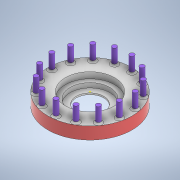
# Autodesk Inventor part: Część1
Saved by Autodesk Inventor 2021 (Build 250183000, 183)
## iProperties
Created: 2022-07-15
Part Number: Część1
Material: Ogólny
Document SubType Name: Modeling
Designer: MicnedSQ
Density: 1 g/cm^3
Appearance: Domyślna
Author: MicnedSQ
## iProperties of the stored document _Drukowanie 3D.ipt
Created: 2022-08-08
Part Number: _Drukowanie 3D
Material: Ogólny
Document SubType Name: Modeling
Designer: MicnedSQ
Density: 1 g/cm^3
Appearance: Domyślna
Author: MicnedSQ
Autodesk Inventor part; units mm, degrees
ref_plane "YZ Plane" through (0, 0, 0) normal (1, 0, 0) x (0, 1, 0)
ref_plane "XZ Plane" through (0, 0, 0) normal (0, 1, 0) x (-1, 0, 0)
ref_plane "XY Plane" through (0, 0, 0) normal (0, 0, 1) x (1, 0, 0)
sketch "Szkic1" plane through (0, 0, 0) normal (0, 1, 0) x (-1, 0, 0)
  circle A0 centre (0, 0) radius 27.5
  dimension "d0" = 55
  constraints: 1 centre point, 1 coincident
  measures "d0" diameter of A0
extrude "Wyciągnięcie proste1" add sketch "Szkic1" along normal blind 8
sketch "Szkic2" plane through (0, 8, 0) normal (0, 1, 0) x (1, 0, 0)
  circle A0 centre (0, 0) radius 25
  circle A1 centre (-25, 0) radius 1.5
  dimension "d3" = 50
  dimension "d4" = 3
  constraints: 1 centre point, 1 coincident, 1 horizontal alignment, 2 other
  measures "d4" diameter of A1
extrude "Wyciągnięcie proste2" add sketch "Szkic2" along normal blind 10 contours A1 A0 | A0 A1 picked at (-24.4967, 0) picked at (-25.4929, -0.0614)
pattern_circular "Szyk kołowy1" count 15 over 360 about axis through (0, 0, 0) along (0, 1, 0) of "Wyciągnięcie proste2"
sketch "Szkic4" plane through (0, 8, 0) normal (0, 1, 0) x (1, 0, 0)
  point P0 (0, 0)
sketch "Szkic5" plane through (0, 8, 0) normal (0, 1, 0) x (1, 0, 0)
  circle A0 centre (0, 0) radius 16.1
  dimension "d13" = 32.2
  constraints: 1 centre point, 1 coincident
  measures "d13" diameter of A0
extrude "Wyciągnięcie proste4" cut sketch "Szkic5" against normal blind 4
sketch "Szkic6" plane through (0, 4, 0) normal (0, 1, 0) x (1, 0, 0)
  circle A0 centre (0, 0) radius 13
  dimension "d16" = 26
  constraints: 1 centre point, 1 coincident
  measures "d16" diameter of A0
extrude "Wyciągnięcie proste5" cut sketch "Szkic6" against normal blind 3
sketch "Szkic9" plane through (0, 0, 0) normal (0, -1, 0) x (1, 0, 0)
  circle A0 centre (24, 0) radius 2.05
  circle A1 centre (0, 24) radius 2.05
  circle A2 centre (-24, 0) radius 2.05
  circle A3 centre (0, -24) radius 2.05
  point P0 (0, 0)
  dimension "d23" = 4.1
  dimension "d26" = 360
  dimension "d30" = 24
  constraints: 4 centre point, 9 other
  measures "d23" diameter of A0
  measures "d30" distance of point (0, 0) A0.centre
extrude "Wyciągnięcie proste7" cut sketch "Szkic9" against normal blind 7
sketch "Szkic10" plane through (0, 1, 0) normal (0, 1, 0) x (1, 0, 0)
  circle A0 centre (0, 0) radius 9
  dimension "d32" = 18
  constraints: 1 centre point, 1 coincident
  measures "d32" diameter of A0
extrude "Wyciągnięcie proste8" cut sketch "Szkic10" against normal blind 4
fillet "Zaokrąglenie1" radius 1 15 edges at (-26.5, 8, 0) (-24.209, 8, -10.7785) (-17.732, 8, -19.6933) (-8.189, 8, -25.203) (2.77, 8, -26.3548) (13.25, 8, -22.9497) (21.439, 8, -15.5763) (25.9209, 8, -5.5097) (25.9209, 8, 5.5097) (21.439, 8, 15.5763) (13.25, 8, 22.9497) (2.77, 8, 26.3548) (-8.189, 8, 25.203) (-17.732, 8, 19.6933) (-24.209, 8, 10.7785)
